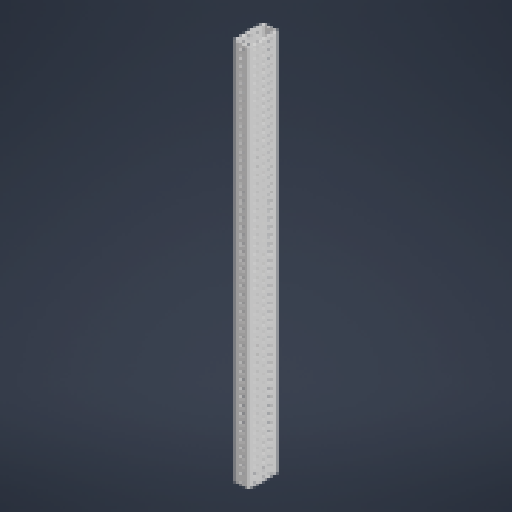
# Autodesk Inventor part: PERFIL 50X25 STEMOS 661,4MM
Saved by Autodesk Inventor 2026 (Build 300175000, 175)
## iProperties
Created: 2026-05-20
Part Number: PERFIL 50X25 STEMOS 661,4MM
Material: Genérico
Document SubType Name: Modeling
Designer: DELL
Density: 1 g/cm^3
Appearance: Padrão
Author: DELL
Autodesk Inventor part; units mm, degrees
ref_plane "YZ Plane" through (0, 0, 0) normal (1, 0, 0) x (0, 1, 0)
ref_plane "XZ Plane" through (0, 0, 0) normal (0, 1, 0) x (-1, 0, 0)
ref_plane "XY Plane" through (0, 0, 0) normal (0, 0, 1) x (1, 0, 0)
sketch "Esboço1" plane through (0, 0, 0) normal (0, 1, 0) x (-1, 0, 0)
  line L0 (0, 0) -> (25.4, 0)
  line L1 (25.4, 0) -> (25.4, -50.8)
  line L2 (25.4, -50.8) -> (0, -50.8)
  line L3 (0, -50.8) -> (0, 0)
  line L4 (23.4, -48.8) -> (23.4, -2)
  line L5 (23.4, -2) -> (2, -2)
  line L6 (2, -2) -> (2, -48.8)
  line L7 (2, -48.8) -> (23.4, -48.8)
  dimension "d0" = 25.4
  dimension "d1" = 50.8
  dimension "d2" = 2
  constraints: 16 end point, 4 parallel, 2 perpendicular, 1 horizontal, 3 other
  measures "d0" distance of L1.end L2.end
  measures "d1" distance of L0.end L1.end
  measures "d2" distance between parallel lines of L1 L4
extrude "Extrusão1" add sketch "Esboço1" along normal blind 1000
sketch "Esboço2" plane through (0, 0, 0) normal (1, 0, 0) x (0, 0, -1)
  circle A0 centre (25.4, 5) radius 2.5
  circle A1 centre (12.7, 5) radius 2.5
  circle A2 centre (38.1, 5) radius 2.5
  line L0 (0, 0) -> (50.8, 0) projected
  line L1 (50.8, 0) -> (50.8, 1000) projected
  dimension "d5" = 5
  dimension "d6" = 5
  dimension "d7" = 5
  dimension "d8" = 5
  dimension "d9" = 5
  dimension "d10" = 5
  dimension "d12" = 25.4
  dimension "d13" = 12.7
  dimension "d14" = 12.7
  constraints: 3 centre point
  measures "d5" diameter of A0
  measures "d6" diameter of A1
  measures "d7" diameter of A2
  measures "d8" distance from line of A1.centre L0
  measures "d9" distance from line of L0 A0.centre
  measures "d10" distance from line of L0 A2.centre
  measures "d12" distance from line of L1 A0.centre
  measures "d13" distance of A2.centre A0.centre
  measures "d14" distance of A1.centre A0.centre
extrude "Extrusão2" cut sketch "Esboço2" against normal blind 1000
sketch "Esboço3" plane through (0, 0, -50.8) normal (0, 0, -1) x (-1, 0, 0)
  circle A0 centre (12.7, 5) radius 2.5
  line L0 (0, 0) -> (25.4, 0) projected
  dimension "d17" = 5
  dimension "d18" = 5
  constraints: 1 centre point
  measures "d17" diameter of A0
  measures "d18" distance from line of L0 A0.centre
extrude "Extrusão3" cut sketch "Esboço3" against normal blind 1000
pattern_linear "Padrão retangular1" count 100 spacing 12.7 along (0, 1, 0) of "Extrusão2", "Extrusão3"
sketch "Esboço4" plane through (0, 0, 0) normal (1, 0, 0) x (0, 0, -1)
  line L0 (50.8, 0) -> (50.8, 1000) projected
  line L1 (0, 0) -> (50.8, 0)
  line L2 (50.8, 0) -> (50.8, 38.1)
  line L3 (50.8, 38.1) -> (0, 38.1)
  line L4 (0, 38.1) -> (0, 0)
  circle A0 centre (38.1, 43.1) radius 2.5 projected
  line L5 (50.8, 1000) -> (0, 1000) projected
  line L6 (0, 1000) -> (50.8, 1000)
  line L7 (50.8, 1000) -> (50.8, 699.5)
  line L8 (50.8, 699.5) -> (0, 699.5)
  line L9 (0, 699.5) -> (0, 1000)
  dimension "d24" = 5
  dimension "d25" = 661.4
  constraints: 16 end point, 4 parallel, 2 horizontal, 2 perpendicular, 2 point on line
  measures "d24" distance from line of A0.centre L3
  measures "d25" distance between parallel lines of L3 L8
extrude "Extrusão4" cut sketch "Esboço4" against normal blind 25.4 contours L1 L4 L3 L0 | L8 L9 L5 L0
equation "\"d9\" = d8"
equation "\"d10\" = d8"
equation "\"d14\" = d13"
